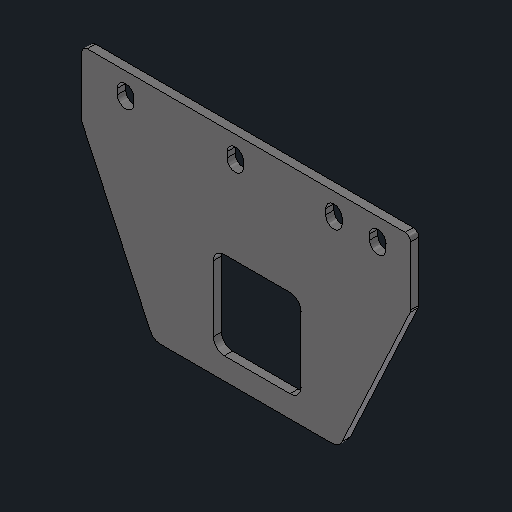
# Autodesk Inventor part: Front Hitch Model-1_Sheet-RH
Saved by Autodesk Inventor 2025.1 (Build 291241000, 241)
## iProperties
RuleStatus: InUse
Created: 2026-02-13
Part Number: Front Hitch Model-1_Sheet-RH
User Status: Released
Material: SS304
Document SubType Name: Sheet Metal
Designer: Desktop -24
Density: 7.99949 g/cm^3
Sheet Metal Rule: 3/8" (3.150 Die)
Appearance: Semi-Polished(1)
AfterDocNew0: Mat. Selection
encoded128: ÌSheet Metal (in)XÎ
Family: SS304
Author: Desktop -24
Revision Number: 0
Autodesk Inventor part; units mm, degrees
ref_plane "YZ Plane" through (0, 0, 0) normal (1, 0, 0) x (0, 1, 0)
ref_plane "XZ Plane" through (0, 0, 0) normal (0, 1, 0) x (-1, 0, 0)
ref_plane "XY Plane" through (0, 0, 0) normal (0, 0, 1) x (1, 0, 0)
sketch "Sketch1" plane through (0, 0, 0) normal (0, 0, 1) x (1, 0, 0)
  line L0 (0, 0) -> (298.0905, 0) construction
  line L1 (381, 254) -> (0, 254)
  line L2 (0, 254) -> (0, 0) construction
  line L3 (0, 254) -> (0, 0) construction
  line L4 (381, 254) -> (381, 177.8)
  line L5 (381, 177.8) -> (298.0905, 0)
  line L6 (0, 254) -> (0, 177.8)
  line L7 (82.9095, 0) -> (0, 177.8)
  line L8 (82.9095, 0) -> (298.0905, 0)
  dimension "d42" = 254
  dimension "d79" = 381
  dimension "d97" = 65
  dimension "d98" = 76.2
  dimension "d99" = 25
  measures "d42" distance of L1.end L0.start
  measures "d79" distance of L1.start L1.end
  measures "d97" angle of L5 L0
  measures "d98" distance of L1.start L4.end
  measures "d99" angle of L2 L7
extrude "Plate1" add sketch "Sketch1" along normal blind 9.525
fillet "Corner Round1" radius 12.7 2 edges at (298.0905, 0, 4.7625) (82.9095, 0, 4.7625)
ref_plane "Work Plane1" through (0, 177.8, -13.208) normal (0, 1, 0) x (1, 0, 0)
sketch "Sketch10" plane through (0, 177.8, 9.525) normal (0, 0, 1) x (1, 0, 0)
  line L0 (342.9, 53.975) -> (342.9, 47.625) construction
  line L1 (333.375, 53.975) -> (333.375, 47.625)
  line L2 (352.425, 47.625) -> (352.425, 53.975)
  arc A0 (352.425, 53.975) -> (333.375, 53.975) centre (342.9, 53.975) ccw
  arc A1 (333.375, 47.625) -> (352.425, 47.625) centre (342.9, 47.625) ccw
  line L3 (50.8, 53.975) -> (50.8, 47.625) construction
  line L4 (41.275, 53.975) -> (41.275, 47.625)
  line L5 (60.325, 47.625) -> (60.325, 53.975)
  arc A2 (60.325, 53.975) -> (41.275, 53.975) centre (50.8, 53.975) ccw
  arc A3 (41.275, 47.625) -> (60.325, 47.625) centre (50.8, 47.625) ccw
  line L6 (0, 76.2) -> (381, 76.2) projected
  line L7 (381, 76.2) -> (381, 0) projected
  arc A4 (282.575, 47.625) -> (301.625, 47.625) centre (292.1, 47.625) ccw
  line L8 (282.575, 53.975) -> (282.575, 47.625)
  arc A5 (301.625, 53.975) -> (282.575, 53.975) centre (292.1, 53.975) ccw
  line L9 (301.625, 47.625) -> (301.625, 53.975)
  arc A6 (187.325, 53.975) -> (168.275, 53.975) centre (177.8, 53.975) ccw
  line L10 (187.325, 47.625) -> (187.325, 53.975)
  arc A7 (168.275, 47.625) -> (187.325, 47.625) centre (177.8, 47.625) ccw
  line L11 (168.275, 53.975) -> (168.275, 47.625)
  line L12 (0, 0) -> (0, 76.2) projected
  point P0 (342.9, 50.8)
  point P1 (50.8, 50.8)
  point P2 (41.275, 50.8)
  point P3 (168.275, 50.8)
  dimension "d83" = 19.05
  dimension "d85" = 6.35
  dimension "d100" = 25.4
  dimension "d101" = 38.1
  dimension "d104" = 50.8
  dimension "d111" = 127
  dimension "d116" = 50.8
  constraints: 24 end point, 16 point on circle, 8 centre point, 8 tangent, 3 midpoint, 3 parallel, 2 horizontal, 2 vertical, 1 equal radius, 1 horizontal alignment, 21 other
  measures "d83" distance between parallel lines of L1 L2
  measures "d85" distance of L0.start L0.end
  measures "d100" distance from line of L6 point (41.275, 50.8)
  measures "d101" distance from line of L7 point (342.9, 50.8)
  measures "d104" distance of L0.end A4.centre
  measures "d111" distance of L3.start A6.centre
  measures "d116" distance from line of point (50.8, 50.8) L12
extrude "Cut4" cut sketch "Sketch10" against normal blind 9.525
sketch "Sketch11" plane through (0, 0, 9.525) normal (0, 0, 1) x (1, 0, 0)
  line L0 (165.1, 127) -> (241.3, 127)
  line L1 (254, 114.3) -> (254, 38.1)
  line L2 (241.3, 25.4) -> (165.1, 25.4)
  line L3 (152.4, 38.1) -> (152.4, 114.3)
  line L4 (152.4, 127) -> (254, 25.4) construction
  line L5 (254, 127) -> (152.4, 25.4) construction
  arc A0 (254, 114.3) -> (241.3, 127) centre (241.3, 114.3) ccw
  arc A1 (165.1, 127) -> (152.4, 114.3) centre (165.1, 114.3) ccw
  arc A2 (152.4, 38.1) -> (165.1, 25.4) centre (165.1, 38.1) ccw
  arc A3 (241.3, 25.4) -> (254, 38.1) centre (241.3, 38.1) ccw
  line L6 (289.9997, 0) -> (0, 0) projected
  line L7 (0, 0) -> (0, 254) projected
  point P0 (203.2, 76.2)
  point P1 (12.7, 0)
  point P2 (0, 12.7)
  point P3 (0, 155.067)
  dimension "d90" = 101.6
  dimension "d91" = 101.6
  dimension "d92" = 12.7
  dimension "d93" = 25.4
  dimension "d94" = 152.4
  constraints: 12 end point, 8 point on circle, 8 point on line, 8 tangent, 4 centre point, 3 equal radius, 2 midpoint, 2 parallel, 1 horizontal, 1 perpendicular
  measures "d90" distance of L5.start L4.end
  measures "d91" distance of L4.end L5.end
  measures "d92" radius of A0
  measures "d93" distance between parallel lines of L6 L2
  measures "d94" distance between parallel lines of L7 L3
extrude "Cut5" cut sketch "Sketch11" against normal blind 9.525
fillet "Corner Round4" radius 6.35 4 edges at (381, 254, 4.7625) (381, 177.8, 4.7625) (0, 254, 4.7625) (0, 177.8, 4.7625)
equation "\"d88\" = Thickness"
equation "\"d95\" = Thickness"
equation "\"d15\" = Thickness"
equation "\"BendReliefWidth\" = Thickness"
equation "\"BendReliefDepth\" = 0.5 * Thickness"
equation "\"CornerReliefSize\" = 4 * Thickness"
equation "\"MinimumRemnant\" = 2 * Thickness"
equation "\"TransitionRadius\" = BendRadius"
equation "\"JacobiRadiusSize\" = Thickness"
equation "\"GapSize\" = Thickness"
equation "\"Thickness\" = 9.525"
equation "\"BendRadius\" = 13.208"
body "Solid1"
